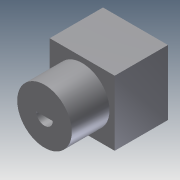
# Autodesk Inventor part: hmodel
Saved by Autodesk Inventor 2011 (Build 150239000, 239)
## iProperties
Created: 2011-12-04
Part Number: hmodel
Document SubType Name: Modeling
Designer: Matthew
Density: 1 g/cm^3
Author: Matthew
Autodesk Inventor part; units mm, degrees
ref_plane "YZ Plane" through (0, 0, 0) normal (1, 0, 0) x (0, 1, 0)
ref_plane "XZ Plane" through (0, 0, 0) normal (0, 1, 0) x (-1, 0, 0)
ref_plane "XY Plane" through (0, 0, 0) normal (0, 0, 1) x (1, 0, 0)
sketch "Sketch1" plane through (0, 0, 0) normal (0, 0, 1) x (1, 0, 0)
  line L0 (-6.6884, 12.6835) -> (43.3116, 12.6835)
  line L1 (43.3116, 12.6835) -> (43.3116, -37.3165)
  line L2 (43.3116, -37.3165) -> (-6.6884, -37.3165)
  line L3 (-6.6884, -37.3165) -> (-6.6884, 12.6835)
  point P0 (0, 0)
  dimension "d0" = 50
  dimension "d1" = 50
  constraints: 8 end point, 2 parallel, 1 horizontal, 1 perpendicular
  measures "d0" distance of L1.end L2.end
  measures "d1" distance of L0.end L1.end
extrude "Extrusion1" add sketch "Sketch1" along normal blind 41
sketch "Sketch2" plane through (0, 0, 41) normal (0, 0, 1) x (1, 0, 0)
  circle A0 centre (18.3116, -12.3165) radius 21
  point P0 (0, 0)
  dimension "d4" = 42
  constraints: 1 centre point
  measures "d4" diameter of A0
extrude "Extrusion2" add sketch "Sketch2" along normal blind 29
sketch "Sketch3" plane through (18.3116, -12.3165, 70) normal (0, 0, 1) x (1, 0, 0)
  circle A0 centre (0, 0) radius 21 projected
  circle A1 centre (0, 0) radius 6.35
  point P0 (-18.3116, 12.3165)
  dimension "d7" = 12.7
  constraints: 1 centre point, 1 coincident
  measures "d7" diameter of A1
extrude "Extrusion3" cut sketch "Sketch3" against normal blind 29 contours A1
sketch "Sketch4" plane through (18.3116, -12.3165, 41) normal (0, 0, 1) x (1, 0, 0)
  circle A0 centre (0, 0) radius 6.35 projected
  point P0 (-18.3116, 12.3165)
extrude "Extrusion4" add sketch "Sketch4" along normal blind 21
sketch "Sketch5" plane through (18.3116, -12.3165, 62) normal (0, 0, 1) x (1, 0, 0)
  circle A0 centre (0, 0) radius 6.35 projected
  point P0 (-18.3116, 12.3165)
extrude "Extrusion5" cut sketch "Sketch5" against normal blind 1
sketch "Sketch6" plane through (18.3116, -12.3165, 61) normal (0, 0, 1) x (1, 0, 0)
  circle A0 centre (0, 0) radius 6.35 projected
  line L0 (-6.35, 0) -> (6.35, 0)
  point P0 (-18.3116, 12.3165)
  constraints: 2 end point, 2 point on circle, 1 horizontal
extrude "Extrusion6" add sketch "Sketch6" along normal blind 8 contours L0 A0 picked at (1.8268, 2.3873)
sketch "Sketch7" plane through (18.3116, -12.3165, 69) normal (0, 0, 1) x (1, 0, 0)
  arc A0 (6.35, 0) -> (-6.35, 0) centre (0, 0) ccw projected
  line L0 (6.35, 0) -> (-6.35, 0) projected
  point P0 (-18.3116, 12.3165)
extrude "Extrusion7" add sketch "Sketch7" along normal blind 1
sketch "Sketch8" plane through (0, 0, 0) normal (0, 0, -1) x (-1, 0, 0)
  line L0 (-43.3116, 12.6835) -> (-38.3116, 12.6835)
  line L1 (-38.3116, 12.6835) -> (-38.3116, 7.6835)
  line L2 (-38.3116, 7.6835) -> (-43.3116, 7.6835)
  line L3 (-43.3116, 7.6835) -> (-43.3116, 12.6835)
  line L4 (6.6884, -37.3165) -> (1.6884, -37.3165)
  line L5 (1.6884, -37.3165) -> (1.6884, -32.3165)
  line L6 (1.6884, -32.3165) -> (6.6884, -32.3165)
  line L7 (6.6884, -32.3165) -> (6.6884, -37.3165)
  line L8 (-38.3116, 7.6835) -> (1.6884, 7.6835)
  line L9 (1.6884, 7.6835) -> (1.6884, -32.3165)
  line L10 (1.6884, -32.3165) -> (-38.3116, -32.3165)
  line L11 (-38.3116, -32.3165) -> (-38.3116, 7.6835)
  circle A0 centre (-38.3116, -32.3165) radius 0.5
  circle A1 centre (1.6884, 7.6835) radius 0.5
  point P0 (0, 0)
  dimension "d18" = 5
  dimension "d19" = 5
  dimension "d20" = 5
  dimension "d21" = 5
  dimension "d22" = 1
  dimension "d23" = 1
  constraints: 24 end point, 6 parallel, 3 horizontal, 3 perpendicular, 2 centre point, 2 coincident
  measures "d18" distance of L1.end L2.end
  measures "d19" distance of L0.end L1.end
  measures "d20" distance of L5.end L6.end
  measures "d21" distance of L4.end L5.end
  measures "d22" diameter of A0
  measures "d23" diameter of A1
extrude "Extrusion8" cut sketch "Sketch8" against normal blind 6 contours A1 L9 L8 | L8 L9 A1 | A0 L10 L11 | L11 L10 A0
body "Solid1"
